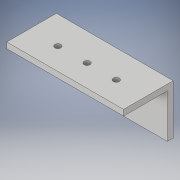
# Autodesk Inventor part: jig proto1
Saved by Autodesk Inventor 2019 (Build 230136000, 136)
## iProperties
Created: 2018-11-25
Part Number: jig proto1
Material: Generic
Document SubType Name: Modeling
Designer: Tiberus
Density: 1 g/cm^3
Appearance: Default
Author: Tiberus
Autodesk Inventor part; units mm, degrees
ref_plane "YZ Plane" through (0, 0, 0) normal (1, 0, 0) x (0, 1, 0)
ref_plane "XZ Plane" through (0, 0, 0) normal (0, 1, 0) x (-1, 0, 0)
ref_plane "XY Plane" through (0, 0, 0) normal (0, 0, 1) x (1, 0, 0)
sketch "Sketch1" plane through (0, 0, 0) normal (0, 1, 0) x (-1, 0, 0)
  line L0 (0, 0) -> (-101.6, 0)
  line L1 (-101.6, 0) -> (-101.6, 38.1)
  line L2 (-101.6, 38.1) -> (0, 38.1)
  line L3 (0, 38.1) -> (0, 0)
  line L4 (0, 19.05) -> (-101.6, 19.05) construction
  line L5 (0, 9.2781) -> (-25.4, 9.2781) construction
  line L6 (-25.4, 9.2781) -> (-50.8, 9.2781) construction
  line L7 (-50.8, 9.2781) -> (-76.2, 9.2781) construction
  line L8 (-76.2, 9.2781) -> (-101.6, 9.2781) construction
  line L9 (-101.6, 9.2781) -> (-101.6, 9.2781) construction
  circle A0 centre (-25.4, 19.05) radius 2.5797
  circle A1 centre (-50.8, 19.05) radius 2.5797
  circle A2 centre (-76.2, 19.05) radius 2.5797
  dimension "d0" = 101.6
  dimension "d1" = 38.1
  dimension "d2" = 25.4
  dimension "d3" = 25.4
  dimension "d4" = 25.4
  dimension "d5" = 25.4
  dimension "d6" = 5.1594
  dimension "d7" = 5.1594
  dimension "d8" = 5.1594
  constraints: 20 end point, 8 point on line, 3 centre point, 3 midpoint, 3 parallel, 1 horizontal, 1 perpendicular
  measures "d0" distance of L1.end L2.end
  measures "d1" distance of L0.end L1.end
  measures "d2" distance of L5.start L5.end
  measures "d3" distance of L5.end L6.end
  measures "d4" distance of L6.end L7.end
  measures "d5" distance of L7.end L8.end
  measures "d6" diameter of A0
  measures "d7" diameter of A1
  measures "d8" diameter of A2
extrude "Extrusion1" add sketch "Sketch1" along normal blind 5.08
sketch "Sketch2" plane through (101.6, 0, 0) normal (0, 0, -1) x (-1, 0, 0)
  line L0 (0, 5.08) -> (101.6, 5.08) projected
  line L1 (101.6, 5.08) -> (0, 5.08)
  line L2 (0, 5.08) -> (0, -38.1)
  line L3 (0, -38.1) -> (101.6, -38.1)
  line L4 (101.6, -38.1) -> (101.6, 5.08)
  point P0 (101.6, 0)
  dimension "d11" = 43.18
  constraints: 8 end point, 2 parallel, 1 horizontal, 1 perpendicular
  measures "d11" distance of L2.end L1.end
extrude "Extrusion2" add sketch "Sketch2" along normal blind 5.08
body "Solid1"
